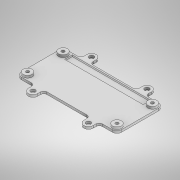
# Autodesk Inventor part: plate
Saved by Autodesk Inventor 2022.2 (Build 262287010, 287A)
## iProperties
Created: 2025-12-31
Part Number: plate
Material: Generic
Document SubType Name: Modeling
Designer: dbstj
Density: 1 g/cm^3
Appearance: Default
Author: dbstj
Autodesk Inventor part; units mm, degrees
ref_plane "YZ Plane" through (0, 0, 0) normal (1, 0, 0) x (0, 1, 0)
ref_plane "XZ Plane" through (0, 0, 0) normal (0, 1, 0) x (-1, 0, 0)
ref_plane "XY Plane" through (0, 0, 0) normal (0, 0, 1) x (1, 0, 0)
sketch "스케치1" plane through (0, 0, 0) normal (0, 1, 0) x (-1, 0, 0)
  line L0 (-29.5, -15) -> (29.5, -15)
  line L1 (32.5, -12) -> (32.5, 12)
  line L2 (29.5, 15) -> (-29.5, 15)
  line L3 (-32.5, 12) -> (-32.5, -12)
  line L4 (-32.5, -15) -> (32.5, 15) construction
  line L5 (32.5, -15) -> (-32.5, 15) construction
  line L6 (-29, -11.5) -> (29, -11.5)
  line L7 (29, -11.5) -> (29, 11.5)
  line L8 (29, 11.5) -> (-29, 11.5)
  line L9 (-29, 11.5) -> (-29, -11.5)
  line L10 (-29, -11.5) -> (29, 11.5) construction
  line L11 (29, -11.5) -> (-29, 11.5) construction
  circle A0 centre (29, 11.5) radius 1
  circle A1 centre (29, -11.5) radius 1
  circle A2 centre (-29, -11.5) radius 1
  circle A3 centre (-29, 11.5) radius 1
  arc A4 (29.5, -15) -> (32.5, -12) centre (29.5, -12) ccw
  arc A5 (-32.5, -12) -> (-29.5, -15) centre (-29.5, -12) ccw
  arc A6 (-29.5, 15) -> (-32.5, 12) centre (-29.5, 12) ccw
  arc A7 (32.5, 12) -> (29.5, 15) centre (29.5, 12) ccw
  point P0 (0, 0)
  point P1 (0, 0)
  point P2 (0, 0)
  point P3 (0, 0)
  point P4 (0, 0)
  dimension "d0" = 65
  dimension "d1" = 30
  dimension "d2" = 58
  dimension "d3" = 23
  dimension "d4" = 2
  dimension "d5" = 2
  dimension "d6" = 2
  dimension "d7" = 2
  dimension "d8" = 3
  constraints: 24 end point, 8 centre point, 8 point on circle, 8 point on line, 8 tangent, 6 coincident, 6 midpoint, 4 parallel, 3 equal radius, 2 horizontal, 2 perpendicular
  measures "d0" distance of L5.end L4.end
  measures "d1" distance of L4.end L5.start
  measures "d2" distance of L11.end L7.end
  measures "d3" distance of L7.end L7.start
  measures "d4" diameter of A0
  measures "d5" diameter of A1
  measures "d6" diameter of A2
  measures "d7" diameter of A3
  measures "d8" radius of A4
extrude "돌출1" add sketch "스케치1" along normal blind 1.5 contours A5 L3 A6 L2 A7 L1 A4 L0 | A2 L9 A3 L8 A0 L7 A1 L6
sketch "스케치2" plane through (0, 1.5, 0) normal (0, 1, 0) x (1, 0, 0)
  circle A0 centre (-29, 11.5) radius 1 projected
  circle A1 centre (-29, 11.5) radius 2.9
  circle A2 centre (29, 11.5) radius 1 projected
  circle A3 centre (29, 11.5) radius 2.9
  circle A4 centre (-29, -11.5) radius 1 projected
  circle A5 centre (-29, -11.5) radius 2.9
  circle A6 centre (29, -11.5) radius 1 projected
  circle A7 centre (29, -11.5) radius 2.9
  point P0 (0, 0)
  dimension "d11" = 5.8
  dimension "d12" = 5.8
  dimension "d13" = 5.8
  dimension "d14" = 5.8
  constraints: 4 centre point, 4 coincident
  measures "d11" diameter of A1
  measures "d12" diameter of A3
  measures "d13" diameter of A5
  measures "d14" diameter of A7
extrude "돌출2" add sketch "스케치2" along normal blind 1.5
sketch "스케치3" plane through (0, 1.5, 0) normal (0, 1, 0) x (1, 0, 0)
  line L0 (-25, 13.5) -> (25, 13.5)
  line L1 (25, 13.5) -> (25, 9.5)
  line L2 (25, 9.5) -> (-25, 9.5)
  line L3 (-25, 9.5) -> (-25, 13.5)
  line L4 (-25, 13.5) -> (25, 9.5) construction
  line L5 (25, 13.5) -> (-25, 9.5) construction
  line L6 (29.5, 15) -> (-29.5, 15) projected
  circle A0 centre (-29, 11.5) radius 1 projected
  point P0 (0, 0)
  point P1 (0, 11.5)
  point P2 (0, 11.5)
  point P3 (0, 11.5)
  dimension "d17" = 50
  dimension "d18" = 4
  dimension "d19" = 3.5
  dimension "d20" = 29
  constraints: 12 end point, 4 midpoint, 2 parallel, 1 horizontal, 1 perpendicular
  measures "d17" distance of L1.end L2.end
  measures "d18" distance of L0.end L1.end
  measures "d19" distance from line of L6 point (0, 11.5)
  measures "d20" distance of A0.centre point (0, 11.5)
extrude "돌출3" cut sketch "스케치3" against normal blind 0.5 contours L0 L1 L2 L3
chamfer "모따기1" distance 0.5 angle 45 4 edges at (25, 1.5, -11.5) (0, 1.5, -13.5) (0, 1.5, -9.5) (-25, 1.5, -11.5)
sketch "스케치4" plane through (0, 0, 0) normal (0, -1, 0) x (1, 0, 0)
  circle A0 centre (-29, 11.5) radius 1 projected
  circle A1 centre (-29, 11.5) radius 2
  circle A2 centre (29, 11.5) radius 1 projected
  circle A3 centre (29, 11.5) radius 2
  circle A4 centre (29, -11.5) radius 1 projected
  circle A5 centre (29, -11.5) radius 2
  circle A6 centre (-29, -11.5) radius 1 projected
  circle A7 centre (-29, -11.5) radius 2
  point P0 (0, 0)
  dimension "d26" = 4
  dimension "d27" = 4
  dimension "d28" = 4
  dimension "d29" = 4
  constraints: 4 centre point, 4 coincident
  measures "d26" diameter of A1
  measures "d27" diameter of A3
  measures "d28" diameter of A5
  measures "d29" diameter of A7
extrude "돌출4" cut sketch "스케치4" against normal blind 1
fillet "모깎기1" radius 0.5 4 edges at (-31, 0, 11.5) (27, 0, 11.5) (27, 0, -11.5) (-31, 0, -11.5)
sketch "스케치5" plane through (0, 1.5, 0) normal (0, 1, 0) x (1, 0, 0)
  line L0 (-18, -19) -> (18, -19)
  line L1 (18, -19) -> (18, 19)
  line L2 (18, 19) -> (-18, 19)
  line L3 (-18, 19) -> (-18, -19)
  line L4 (-18, -19) -> (18, 19) construction
  line L5 (18, -19) -> (-18, 19) construction
  circle A0 centre (-18, 19) radius 1.5
  circle A1 centre (18, 19) radius 1.5
  circle A2 centre (-18, -19) radius 1.5
  circle A3 centre (18, -19) radius 1.5
  circle A4 centre (-18, -19) radius 3
  circle A5 centre (18, -19) radius 3
  circle A6 centre (18, 19) radius 3
  circle A7 centre (-18, 19) radius 3
  line L6 (29.5, 15) -> (-29.5, 15) projected
  line L7 (-29.5, -15) -> (29.5, -15) projected
  line L8 (-21, -19) -> (-21, -15)
  line L9 (-15, -19) -> (-15, -15)
  line L10 (15, -19) -> (15, -15)
  line L11 (21, -19) -> (21, -15)
  line L12 (21, 19) -> (21, 15)
  line L13 (29.5, 15) -> (-29.5, 15) projected
  line L14 (15, 19) -> (15, 15)
  line L15 (-15, 19) -> (-15, 15)
  line L16 (-21, 19) -> (-21, 15)
  point P0 (0, 0)
  dimension "d33" = 36
  dimension "d34" = 38
  dimension "d35" = 3
  dimension "d36" = 3
  dimension "d37" = 3
  dimension "d38" = 3
  dimension "d42" = 6
  dimension "d43" = 6
  constraints: 28 end point, 16 point on line, 8 centre point, 8 coincident, 8 point on circle, 7 perpendicular, 4 tangent, 2 midpoint, 2 parallel, 1 horizontal
  measures "d33" distance of L2.end L1.end
  measures "d34" distance of L1.end L0.end
  measures "d35" diameter of A0
  measures "d36" diameter of A1
  measures "d37" diameter of A2
  measures "d38" diameter of A3
  measures "d42" diameter of A7
  measures "d43" diameter of A6
extrude "돌출5" add sketch "스케치5" against normal up to surface (1.5 mm away) contours A2 L3 A4 L0 | L0 A4 L3 A2 | A4 L3 L7 L9 | A4 L8 L7 L3 | A5 L1 A3 L0 | L0 A3 L1 A5 | L10 L7 L1 A5 | A5 L1 L7 L11 | L6 L16 A7 L3 | L3 A7 L15 L6 | A7 L2 A0 L3 | L3 A0 L2 A7 | L6 L14 A6 L1 | L1 A6 L12 L6 | A6 L2 A1 L1 | L1 A1 L2 A6
fillet "모깎기2" radius 2 8 edges at (-21, 0.75, 15) (15, 0.75, 15) (21, 0.75, 15) (-15, 0.75, 15) (-15, 0.75, -15) (21, 0.75, -15) (-21, 0.75, -15) (15, 0.75, -15)
equation "\"d4\" = d5"
equation "\"d6\" = d5"
equation "\"d7\" = d5"
equation "\"d27\" = d26"
equation "\"d28\" = d26"
equation "\"d29\" = d26"
